Autodesk Inventor part; units mm, degrees
(part 2 of 2)
  line L262 (13.6018, -17.5742) -> (13.2961, -17.2686)
  spline S264 degree 2 poles (13.2961, -17.2686) (13.3171, -17.2092) (13.3852, -17.0328) (13.4219, -16.9716) knots 0 0 0 1 2 2 2
  spline S265 degree 2 poles (13.4219, -16.9716) (13.4708, -16.8808) (13.5599, -16.7498) (13.6454, -16.6642) knots 0 0 0 1 2 2 2
  spline S266 degree 2 poles (12.2779, -18.0318) (12.4455, -17.8641) (12.8263, -17.6895) (13.0306, -17.6947) knots 0 0 0 1 2 2 2
  spline S267 degree 2 poles (13.0306, -17.6947) (13.2332, -17.6982) (13.6612, -17.906) (13.8742, -18.1191) knots 0 0 0 1 2 2 2
  spline S268 degree 2 poles (13.8742, -18.1191) (14.0873, -18.3322) (14.2847, -18.7566) (14.2934, -18.9575) knots 0 0 0 1 2 2 2
  spline S269 degree 2 poles (14.2934, -18.9575) (14.3039, -19.1601) (14.1327, -19.5583) (13.9686, -19.7225) knots 0 0 0 1 2 2 2
  spline S270 degree 2 poles (13.9686, -19.7225) (13.8358, -19.8552) (13.5127, -20.0281) (13.3677, -20.0753) knots 0 0 0 1 2 2 2
  line L263 (13.3677, -20.0753) -> (13.0621, -19.7696)
  line L264 (13.0621, -19.7696) -> (13.0778, -19.7539)
  spline S271 degree 2 poles (13.0778, -19.7539) (13.1319, -19.7487) (13.2856, -19.7207) (13.3835, -19.6893) knots 0 0 0 1 2 2 2
  spline S272 degree 2 poles (13.3835, -19.6893) (13.469, -19.6596) (13.6664, -19.5496) (13.7363, -19.4797) knots 0 0 0 1 2 2 2
  spline S273 degree 2 poles (13.7363, -19.4797) (13.9476, -19.2684) (13.8847, -18.692) (13.593, -18.4003) knots 0 0 0 1 2 2 2
  spline S274 degree 2 poles (13.593, -18.4003) (13.3084, -18.1156) (12.7407, -18.044) (12.5207, -18.2641) knots 0 0 0 1 2 2 2
  spline S275 degree 2 poles (12.5207, -18.2641) (12.3879, -18.3968) (12.2569, -18.7479) (12.2499, -18.926) knots 0 0 0 1 2 2 2
  line L265 (12.2499, -18.926) -> (12.2342, -18.9418)
  line L266 (12.2342, -18.9418) -> (11.9286, -18.6361)
  spline S276 degree 2 poles (11.9286, -18.6361) (11.9495, -18.5767) (12.0176, -18.4003) (12.0543, -18.3392) knots 0 0 0 1 2 2 2
  spline S277 degree 2 poles (12.0543, -18.3392) (12.1032, -18.2484) (12.1923, -18.1174) (12.2779, -18.0318) knots 0 0 0 1 2 2 2
  line L267 (11.312, -19.071) -> (11.5845, -18.7985)
  line L268 (11.5845, -18.7985) -> (13.2018, -20.4159)
  line L269 (13.2018, -20.4159) -> (12.9293, -20.6883)
  line L270 (12.9293, -20.6883) -> (11.312, -19.071)
  line L271 (13.1791, -20.9765) -> (13.4882, -20.6674)
  line L272 (13.4882, -20.6674) -> (13.7712, -20.9503)
  line L273 (13.7712, -20.9503) -> (13.462, -21.2595)
  line L274 (13.462, -21.2595) -> (13.1791, -20.9765)
  spline S278 degree 2 poles (10.3916, -21.6088) (9.9829, -21.2001) (9.9305, -20.3617) (10.2588, -20.0334) knots 0 0 0 1 2 2 2
  spline S279 degree 2 poles (10.2588, -20.0334) (10.5959, -19.6963) (11.4413, -19.7696) (11.836, -20.1644) knots 0 0 0 1 2 2 2
  spline S280 degree 2 poles (11.836, -20.1644) (12.2412, -20.5696) (12.2919, -21.4166) (11.967, -21.7415) knots 0 0 0 1 2 2 2
  spline S281 degree 2 poles (11.967, -21.7415) (11.6386, -22.0699) (10.7985, -22.0157) (10.3916, -21.6088) knots 0 0 0 1 2 2 2
  spline S282 degree 2 poles (10.6728, -21.3276) (10.9872, -21.642) (11.5216, -21.7188) (11.7329, -21.5075) knots 0 0 0 1 2 2 2
  spline S283 degree 2 poles (11.7329, -21.5075) (11.9443, -21.2961) (11.8692, -20.7599) (11.5548, -20.4456) knots 0 0 0 1 2 2 2
  spline S284 degree 2 poles (11.5548, -20.4456) (11.2492, -20.1399) (10.7042, -20.0561) (10.4929, -20.2674) knots 0 0 0 1 2 2 2
  spline S285 degree 2 poles (10.4929, -20.2674) (10.2833, -20.477) (10.3619, -21.0167) (10.6728, -21.3276) knots 0 0 0 1 2 2 2
  line L275 (14.7087, -8.5772) -> (15.9575, -7.3284)
  line L276 (15.9575, -7.3284) -> (18.1127, -9.4837)
  line L277 (18.1127, -9.4837) -> (17.8263, -9.7701)
  line L278 (17.8263, -9.7701) -> (15.926, -7.8699)
  line L279 (15.926, -7.8699) -> (14.9637, -8.8322)
  line L280 (14.9637, -8.8322) -> (14.7087, -8.5772)
  spline S286 degree 2 poles (13.7655, -9.447) (14.1533, -9.0593) (15.0143, -9.068) (15.416, -9.4697) knots 0 0 0 1 2 2 2
  spline S287 degree 2 poles (15.416, -9.4697) (15.8107, -9.8644) (15.8649, -10.7464) (15.5313, -11.08) knots 0 0 0 1 2 2 2
  spline S288 degree 2 poles (15.5313, -11.08) (15.3811, -11.2302) (15.0615, -11.3752) (14.8833, -11.3682) knots 0 0 0 1 2 2 2
  spline S289 degree 2 poles (14.8833, -11.3682) (14.7034, -11.363) (14.3436, -11.1883) (14.1498, -10.9945) knots 0 0 0 1 2 2 2
  line L281 (14.1498, -10.9945) -> (14.0013, -10.846)
  line L282 (14.0013, -10.846) -> (15.1209, -9.7265)
  spline S290 degree 2 poles (15.1209, -9.7265) (14.8397, -9.4453) (14.258, -9.4295) (14.0065, -9.681) knots 0 0 0 1 2 2 2
  spline S291 degree 2 poles (14.0065, -9.681) (13.9175, -9.7701) (13.7847, -9.9832) (13.7463, -10.0845) knots 0 0 0 1 2 2 2
  spline S292 degree 2 poles (13.7463, -10.0845) (13.7079, -10.1928) (13.6677, -10.3552) (13.6625, -10.4163) knots 0 0 0 1 2 2 2
  line L283 (13.6625, -10.4163) -> (13.6468, -10.4321)
  line L284 (13.6468, -10.4321) -> (13.3498, -10.1351)
  spline S293 degree 2 poles (13.3498, -10.1351) (13.3778, -10.0688) (13.4651, -9.8697) (13.5053, -9.7981) knots 0 0 0 1 2 2 2
  spline S294 degree 2 poles (13.5053, -9.7981) (13.5612, -9.6968) (13.6677, -9.5448) (13.7655, -9.447) knots 0 0 0 1 2 2 2
  spline S295 degree 2 poles (14.4746, -10.7884) (14.5881, -10.8949) (14.7942, -11.0102) (14.8921, -11.0207) knots 0 0 0 1 2 2 2
  spline S296 degree 2 poles (14.8921, -11.0207) (15.0003, -11.0346) (15.2134, -10.9508) (15.3235, -10.8408) knots 0 0 0 1 2 2 2
  spline S297 degree 2 poles (15.3235, -10.8408) (15.4317, -10.7325) (15.5191, -10.5159) (15.5191, -10.3901) knots 0 0 0 1 2 2 2
  spline S298 degree 2 poles (15.5191, -10.3901) (15.5156, -10.2644) (15.423, -10.0461) (15.3287, -9.9343) knots 0 0 0 1 2 2 2
  line L285 (15.3287, -9.9343) -> (14.4746, -10.7884)
  spline S299 degree 2 poles (12.4242, -12.479) (12.0155, -12.0703) (11.9631, -11.232) (12.2914, -10.9036) knots 0 0 0 1 2 2 2
  spline S300 degree 2 poles (12.2914, -10.9036) (12.6285, -10.5665) (13.4738, -10.6399) (13.8686, -11.0346) knots 0 0 0 1 2 2 2
  spline S301 degree 2 poles (13.8686, -11.0346) (14.2738, -11.4398) (14.3244, -12.2869) (13.9996, -12.6118) knots 0 0 0 1 2 2 2
  spline S302 degree 2 poles (13.9996, -12.6118) (13.6712, -12.9401) (12.8311, -12.886) (12.4242, -12.479) knots 0 0 0 1 2 2 2
  spline S303 degree 2 poles (12.7054, -12.1978) (13.0197, -12.5122) (13.5542, -12.5891) (13.7655, -12.3777) knots 0 0 0 1 2 2 2
  spline S304 degree 2 poles (13.7655, -12.3777) (13.9769, -12.1664) (13.9017, -11.6302) (13.5874, -11.3158) knots 0 0 0 1 2 2 2
  spline S305 degree 2 poles (13.5874, -11.3158) (13.2817, -11.0102) (12.7368, -10.9263) (12.5255, -11.1377) knots 0 0 0 1 2 2 2
  spline S306 degree 2 poles (12.5255, -11.1377) (12.3159, -11.3473) (12.3945, -11.887) (12.7054, -12.1978) knots 0 0 0 1 2 2 2
  line L286 (10.0663, -13.2196) -> (10.3388, -12.9471)
  line L287 (10.3388, -12.9471) -> (11.2609, -13.8693)
  spline S307 degree 2 poles (11.2609, -13.8693) (11.3727, -13.9811) (11.5858, -14.1522) (11.6749, -14.1784) knots 0 0 0 1 2 2 2
  spline S308 degree 2 poles (11.6749, -14.1784) (11.7692, -14.2064) (11.9473, -14.147) (12.0486, -14.0457) knots 0 0 0 1 2 2 2
  spline S309 degree 2 poles (12.0486, -14.0457) (12.1499, -13.9444) (12.2565, -13.6213) (12.2722, -13.4309) knots 0 0 0 1 2 2 2
  line L288 (12.2722, -13.4309) -> (11.0636, -12.2223)
  line L289 (11.0636, -12.2223) -> (11.336, -11.9498)
  line L290 (11.336, -11.9498) -> (12.9534, -13.5671)
  line L291 (12.9534, -13.5671) -> (12.6809, -13.8396)
  line L292 (12.6809, -13.8396) -> (12.501, -13.6597)
  spline S310 degree 2 poles (12.501, -13.6597) (12.4888, -13.892) (12.3683, -14.2431) (12.2355, -14.3758) knots 0 0 0 1 2 2 2
  spline S311 degree 2 poles (12.2355, -14.3758) (11.998, -14.6133) (11.4146, -14.5679) (11.116, -14.2693) knots 0 0 0 1 2 2 2
  line L293 (11.116, -14.2693) -> (10.0663, -13.2196)
  spline S312 degree 2 poles (8.9537, -14.6745) (8.9625, -14.6168) (8.9869, -14.4177) (9.0131, -14.3391) knots 0 0 0 1 2 2 2
  spline S313 degree 2 poles (9.0131, -14.3391) (9.0463, -14.2291) (9.1406, -14.0544) (9.2629, -13.9322) knots 0 0 0 1 2 2 2
  spline S314 degree 2 poles (9.2629, -13.9322) (9.3624, -13.8326) (9.6174, -13.7278) (9.7537, -13.7278) knots 0 0 0 1 2 2 2
  spline S315 degree 2 poles (9.7537, -13.7278) (9.8846, -13.7296) (10.1589, -13.8466) (10.2671, -13.9549) knots 0 0 0 1 2 2 2
  spline S316 degree 2 poles (10.2671, -13.9549) (10.4348, -14.1226) (10.5309, -14.5016) (10.4453, -14.7234) knots 0 0 0 1 2 2 2
  spline S317 degree 2 poles (10.4453, -14.7234) (10.3719, -14.9225) (10.0488, -15.3399) (9.8462, -15.567) knots 0 0 0 1 2 2 2
  line L294 (9.8462, -15.567) -> (9.8986, -15.6194)
  spline S318 degree 2 poles (9.8986, -15.6194) (9.9929, -15.7137) (10.1676, -15.7731) (10.2532, -15.7538) knots 0 0 0 1 2 2 2
  spline S319 degree 2 poles (10.2532, -15.7538) (10.3388, -15.7346) (10.5099, -15.6054) (10.5903, -15.525) knots 0 0 0 1 2 2 2
  spline S320 degree 2 poles (10.5903, -15.525) (10.6846, -15.4307) (10.8837, -15.1198) (10.957, -14.9382) knots 0 0 0 1 2 2 2
  line L295 (10.957, -14.9382) -> (10.9728, -14.9225)
  line L296 (10.9728, -14.9225) -> (11.2505, -15.2002)
  spline S321 degree 2 poles (11.2505, -15.2002) (11.1963, -15.2962) (10.9675, -15.6298) (10.8295, -15.7678) knots 0 0 0 1 2 2 2
  spline S322 degree 2 poles (10.8295, -15.7678) (10.6619, -15.9355) (10.3807, -16.1119) (10.2217, -16.1346) knots 0 0 0 1 2 2 2
  spline S323 degree 2 poles (10.2217, -16.1346) (10.0663, -16.1573) (9.7676, -16.0333) (9.6157, -15.8813) knots 0 0 0 1 2 2 2
  line L297 (9.6157, -15.8813) -> (8.5101, -14.7758)
  line L298 (8.5101, -14.7758) -> (8.7826, -14.5033)
  line L299 (8.7826, -14.5033) -> (8.9537, -14.6745)
  line L300 (9.1808, -14.9015) -> (9.6297, -15.3504)
  spline S324 degree 2 poles (9.6297, -15.3504) (9.7187, -15.2439) (9.9842, -14.919) (10.0488, -14.7985) knots 0 0 0 1 2 2 2
  spline S325 degree 2 poles (10.0488, -14.7985) (10.1239, -14.657) (10.1274, -14.3776) (10.0052, -14.2553) knots 0 0 0 1 2 2 2
  spline S326 degree 2 poles (10.0052, -14.2553) (9.8654, -14.1156) (9.5668, -14.1313) (9.4166, -14.2815) knots 0 0 0 1 2 2 2
  spline S327 degree 2 poles (9.4166, -14.2815) (9.2891, -14.409) (9.1895, -14.7286) (9.1808, -14.9015) knots 0 0 0 1 2 2 2
  line L301 (8.5957, -17.3415) -> (8.6097, -17.3275)
  spline S328 degree 2 poles (8.6097, -17.3275) (8.6498, -17.3048) (8.7214, -17.2402) (8.7686, -17.193) knots 0 0 0 1 2 2 2
  spline S329 degree 2 poles (8.7686, -17.193) (8.8786, -17.083) (8.9991, -16.7703) (9.0026, -16.5782) knots 0 0 0 1 2 2 2
  line L302 (9.0026, -16.5782) -> (7.8551, -15.4307)
  line L303 (7.8551, -15.4307) -> (8.1276, -15.1583)
  line L304 (8.1276, -15.1583) -> (9.7449, -16.7756)
  line L305 (9.7449, -16.7756) -> (9.4725, -17.0481)
  line L306 (9.4725, -17.0481) -> (9.2314, -16.807)
  spline S330 degree 2 poles (9.2314, -16.807) (9.2157, -17.0882) (9.1022, -17.4183) (8.9974, -17.5231) knots 0 0 0 1 2 2 2
  spline S331 degree 2 poles (8.9974, -17.5231) (8.9555, -17.565) (8.9101, -17.6035) (8.8786, -17.6244) knots 0 0 0 1 2 2 2
  line L307 (8.8786, -17.6244) -> (8.5957, -17.3415)
  line L308 (5.8152, -17.4707) -> (6.0876, -17.1983)
  line L309 (6.0876, -17.1983) -> (6.2518, -17.3624)
  spline S332 degree 2 poles (6.2518, -17.3624) (6.2623, -17.2472) (6.285, -17.0847) (6.3182, -16.9922) knots 0 0 0 1 2 2 2
  spline S333 degree 2 poles (6.3182, -16.9922) (6.3479, -16.9066) (6.4422, -16.7529) (6.5243, -16.6708) knots 0 0 0 1 2 2 2
  spline S334 degree 2 poles (6.5243, -16.6708) (6.657, -16.5381) (6.9906, -16.4245) (7.1757, -16.4525) knots 0 0 0 1 2 2 2
  spline S335 degree 2 poles (7.1757, -16.4525) (7.3609, -16.4804) (7.7626, -16.7075) (7.9669, -16.9118) knots 0 0 0 1 2 2 2
  spline S336 degree 2 poles (7.9669, -16.9118) (8.18, -17.1249) (8.3809, -17.5458) (8.4018, -17.7589) knots 0 0 0 1 2 2 2
  spline S337 degree 2 poles (8.4018, -17.7589) (8.4175, -17.9528) (8.2883, -18.323) (8.1503, -18.461) knots 0 0 0 1 2 2 2
  spline S338 degree 2 poles (8.1503, -18.461) (8.0298, -18.5815) (7.7958, -18.7073) (7.6403, -18.751) knots 0 0 0 1 2 2 2
  line L310 (7.6403, -18.751) -> (8.3389, -19.4496)
  line L311 (8.3389, -19.4496) -> (8.0665, -19.722)
  line L312 (8.0665, -19.722) -> (5.8152, -17.4707)
  line L313 (6.4806, -17.5912) -> (7.415, -18.5256)
  spline S339 degree 2 poles (7.415, -18.5256) (7.5652, -18.4732) (7.7626, -18.3492) (7.8551, -18.2567) knots 0 0 0 1 2 2 2
  spline S340 degree 2 poles (7.8551, -18.2567) (8.0647, -18.0471) (7.9879, -17.4952) (7.691, -17.1983) knots 0 0 0 1 2 2 2
  spline S341 degree 2 poles (7.691, -17.1983) (7.4045, -16.9118) (6.9207, -16.7913) (6.7199, -16.9922) knots 0 0 0 1 2 2 2
  spline S342 degree 2 poles (6.7199, -16.9922) (6.6133, -17.0987) (6.4946, -17.4131) (6.4806, -17.5912) knots 0 0 0 1 2 2 2
  spline S343 degree 2 poles (4.9, -20.0032) (4.4913, -19.5945) (4.4389, -18.7562) (4.7672, -18.4278) knots 0 0 0 1 2 2 2
  spline S344 degree 2 poles (4.7672, -18.4278) (5.1043, -18.0908) (5.9496, -18.1641) (6.3444, -18.5588) knots 0 0 0 1 2 2 2
  spline S345 degree 2 poles (6.3444, -18.5588) (6.7496, -18.964) (6.8002, -19.8111) (6.4754, -20.136) knots 0 0 0 1 2 2 2
  spline S346 degree 2 poles (6.4754, -20.136) (6.147, -20.4643) (5.3069, -20.4102) (4.9, -20.0032) knots 0 0 0 1 2 2 2
  spline S347 degree 2 poles (5.1811, -19.722) (5.4955, -20.0364) (6.03, -20.1133) (6.2413, -19.9019) knots 0 0 0 1 2 2 2
  spline S348 degree 2 poles (6.2413, -19.9019) (6.4526, -19.6906) (6.3775, -19.1544) (6.0632, -18.84) knots 0 0 0 1 2 2 2
  spline S349 degree 2 poles (6.0632, -18.84) (5.7575, -18.5344) (5.2126, -18.4505) (5.0013, -18.6619) knots 0 0 0 1 2 2 2
  spline S350 degree 2 poles (5.0013, -18.6619) (4.7917, -18.8715) (4.8703, -19.4112) (5.1811, -19.722) knots 0 0 0 1 2 2 2
  line L314 (-17.3745, -18.836) -> (-14.477, -17.4231)
  line L315 (-14.477, -17.4231) -> (-14.1679, -17.7322)
  line L316 (-14.1679, -17.7322) -> (-15.5808, -20.6297)
  line L317 (-15.5808, -20.6297) -> (-15.8882, -20.3224)
  line L318 (-15.8882, -20.3224) -> (-14.6953, -17.9348)
  line L319 (-14.6953, -17.9348) -> (-17.0829, -19.1277)
  line L320 (-17.0829, -19.1277) -> (-17.3745, -18.836)
  line L321 (-15.6821, -16.2179) -> (-15.4097, -16.4904)
  line L322 (-15.4097, -16.4904) -> (-17.027, -18.1077)
  line L323 (-17.027, -18.1077) -> (-17.2994, -17.8352)
  line L324 (-17.2994, -17.8352) -> (-15.6821, -16.2179)
  line L325 (-17.5876, -18.085) -> (-17.2785, -18.3941)
  line L326 (-17.2785, -18.3941) -> (-17.5614, -18.6771)
  line L327 (-17.5614, -18.6771) -> (-17.8706, -18.3679)
  line L328 (-17.8706, -18.3679) -> (-17.5876, -18.085)
  spline S351 degree 2 poles (-16.5397, -15.2975) (-16.3179, -15.5193) (-16.3214, -16.0223) (-16.5956, -16.2965) knots 0 0 0 1 2 2 2
  line L329 (-16.5956, -16.2965) -> (-17.4916, -17.1925)
  line L330 (-17.4916, -17.1925) -> (-17.3082, -17.3759)
  line L331 (-17.3082, -17.3759) -> (-17.5335, -17.6012)
  line L332 (-17.5335, -17.6012) -> (-17.7169, -17.4178)
  line L333 (-17.7169, -17.4178) -> (-18.1815, -17.8824)
  line L334 (-18.1815, -17.8824) -> (-18.4539, -17.6099)
  line L335 (-18.4539, -17.6099) -> (-17.9893, -17.1454)
  line L336 (-17.9893, -17.1454) -> (-18.4906, -16.6441)
  line L337 (-18.4906, -16.6441) -> (-18.2653, -16.4188)
  line L338 (-18.2653, -16.4188) -> (-17.764, -16.92)
  line L339 (-17.764, -16.92) -> (-16.9938, -16.1498)
  spline S352 degree 2 poles (-16.9938, -16.1498) (-16.8715, -16.0275) (-16.7458, -15.8843) (-16.7178, -15.797) knots 0 0 0 1 2 2 2
  spline S353 degree 2 poles (-16.7178, -15.797) (-16.6916, -15.7219) (-16.751, -15.5612) (-16.8453, -15.4669) knots 0 0 0 1 2 2 2
  spline S354 degree 2 poles (-16.8453, -15.4669) (-16.9117, -15.4005) (-17.0759, -15.3167) (-17.1161, -15.301) knots 0 0 0 1 2 2 2
  line L340 (-17.1161, -15.301) -> (-17.1318, -15.2853)
  line L341 (-17.1318, -15.2853) -> (-16.8873, -15.0407)
  spline S355 degree 2 poles (-16.8873, -15.0407) (-16.7894, -15.0966) (-16.6078, -15.2294) (-16.5397, -15.2975) knots 0 0 0 1 2 2 2
  spline S356 degree 2 poles (-17.5317, -14.3054) (-17.3099, -14.5272) (-17.3134, -15.0303) (-17.5876, -15.3045) knots 0 0 0 1 2 2 2
  line L342 (-17.5876, -15.3045) -> (-18.4836, -16.2005)
  line L343 (-18.4836, -16.2005) -> (-18.3002, -16.3838)
  line L344 (-18.3002, -16.3838) -> (-18.5255, -16.6092)
  line L345 (-18.5255, -16.6092) -> (-18.7089, -16.4258)
  line L346 (-18.7089, -16.4258) -> (-19.1735, -16.8904)
  line L347 (-19.1735, -16.8904) -> (-19.446, -16.6179)
  line L348 (-19.446, -16.6179) -> (-18.9814, -16.1533)
  line L349 (-18.9814, -16.1533) -> (-19.4827, -15.652)
  line L350 (-19.4827, -15.652) -> (-19.2573, -15.4267)
  line L351 (-19.2573, -15.4267) -> (-18.7561, -15.928)
  line L352 (-18.7561, -15.928) -> (-17.9858, -15.1578)
  spline S357 degree 2 poles (-17.9858, -15.1578) (-17.8636, -15.0355) (-17.7378, -14.8923) (-17.7099, -14.805) knots 0 0 0 1 2 2 2
  spline S358 degree 2 poles (-17.7099, -14.805) (-17.6837, -14.7299) (-17.7431, -14.5692) (-17.8374, -14.4749) knots 0 0 0 1 2 2 2
  spline S359 degree 2 poles (-17.8374, -14.4749) (-17.9038, -14.4085) (-18.0679, -14.3246) (-18.1081, -14.3089) knots 0 0 0 1 2 2 2
  line L353 (-18.1081, -14.3089) -> (-18.1238, -14.2932)
  line L354 (-18.1238, -14.2932) -> (-17.8793, -14.0487)
  spline S360 degree 2 poles (-17.8793, -14.0487) (-17.7815, -14.1046) (-17.5999, -14.2373) (-17.5317, -14.3054) knots 0 0 0 1 2 2 2
  line L355 (-18.3439, -13.5562) -> (-18.0714, -13.8286)
  line L356 (-18.0714, -13.8286) -> (-19.6887, -15.4459)
  line L357 (-19.6887, -15.4459) -> (-19.9612, -15.1735)
  line L358 (-19.9612, -15.1735) -> (-18.3439, -13.5562)
  line L359 (-20.2494, -15.4232) -> (-19.9403, -15.7324)
  line L360 (-19.9403, -15.7324) -> (-20.2232, -16.0153)
  line L361 (-20.2232, -16.0153) -> (-20.5323, -15.7062)
  line L362 (-20.5323, -15.7062) -> (-20.2494, -15.4232)
  spline S361 degree 2 poles (-8.1645, -16.5546) (-7.9357, -16.7834) (-7.6964, -17.3021) (-7.7016, -17.5798) knots 0 0 0 1 2 2 2
  spline S362 degree 2 poles (-7.7016, -17.5798) (-7.7086, -17.8593) (-7.9863, -18.4269) (-8.2605, -18.7011) knots 0 0 0 1 2 2 2
  spline S363 degree 2 poles (-8.2605, -18.7011) (-8.5208, -18.9613) (-9.0797, -19.2268) (-9.3626, -19.2373) knots 0 0 0 1 2 2 2
  spline S364 degree 2 poles (-9.3626, -19.2373) (-9.6351, -19.2478) (-10.173, -19.0172) (-10.4018, -18.7884) knots 0 0 0 1 2 2 2
  spline S365 degree 2 poles (-10.4018, -18.7884) (-10.5119, -18.6784) (-10.6795, -18.4479) (-10.7424, -18.3291) knots 0 0 0 1 2 2 2
  spline S366 degree 2 poles (-10.7424, -18.3291) (-10.7948, -18.2348) (-10.8961, -17.9798) (-10.9223, -17.8977) knots 0 0 0 1 2 2 2
  line L363 (-10.9223, -17.8977) -> (-10.5765, -17.5519)
  line L364 (-10.5765, -17.5519) -> (-10.552, -17.5763)
  spline S367 degree 2 poles (-10.552, -17.5763) (-10.545, -17.6776) (-10.5171, -17.8767) (-10.4612, -18.0304) knots 0 0 0 1 2 2 2
  spline S368 degree 2 poles (-10.4612, -18.0304) (-10.4175, -18.1614) (-10.2499, -18.4444) (-10.1206, -18.5736) knots 0 0 0 1 2 2 2
  spline S369 degree 2 poles (-10.1206, -18.5736) (-9.8097, -18.8845) (-8.9574, -18.8007) (-8.5679, -18.4112) knots 0 0 0 1 2 2 2
  spline S370 degree 2 poles (-8.5679, -18.4112) (-8.3514, -18.1946) (-8.1278, -17.7684) (-8.1121, -17.5606) knots 0 0 0 1 2 2 2
  spline S371 degree 2 poles (-8.1121, -17.5606) (-8.0929, -17.3563) (-8.2378, -16.9772) (-8.402, -16.8131) knots 0 0 0 1 2 2 2
  spline S372 degree 2 poles (-8.402, -16.8131) (-8.5225, -16.6926) (-8.7985, -16.4865) (-8.9155, -16.4393) knots 0 0 0 1 2 2 2
  line L365 (-8.9155, -16.4393) -> (-9.4727, -16.9965)
  line L366 (-9.4727, -16.9965) -> (-8.9731, -17.496)
  line L367 (-8.9731, -17.496) -> (-9.2246, -17.7475)
  line L368 (-9.2246, -17.7475) -> (-10.0071, -16.965)
  line L369 (-10.0071, -16.965) -> (-9.0657, -16.0236)
  spline S373 degree 2 poles (-9.0657, -16.0236) (-8.9871, -16.0533) (-8.7269, -16.1633) (-8.6256, -16.2192) knots 0 0 0 1 2 2 2
  spline S374 degree 2 poles (-8.6256, -16.2192) (-8.4876, -16.2943) (-8.285, -16.4341) (-8.1645, -16.5546) knots 0 0 0 1 2 2 2
  spline S375 degree 2 poles (-10.3337, -14.8115) (-10.2761, -14.8202) (-10.077, -14.8447) (-9.9984, -14.8709) knots 0 0 0 1 2 2 2
  spline S376 degree 2 poles (-9.9984, -14.8709) (-9.8883, -14.9041) (-9.7137, -14.9984) (-9.5914, -15.1206) knots 0 0 0 1 2 2 2
  spline S377 degree 2 poles (-9.5914, -15.1206) (-9.4919, -15.2202) (-9.3871, -15.4752) (-9.3871, -15.6114) knots 0 0 0 1 2 2 2
  spline S378 degree 2 poles (-9.3871, -15.6114) (-9.3888, -15.7424) (-9.5058, -16.0166) (-9.6141, -16.1249) knots 0 0 0 1 2 2 2
  spline S379 degree 2 poles (-9.6141, -16.1249) (-9.7818, -16.2926) (-10.1608, -16.3887) (-10.3826, -16.3031) knots 0 0 0 1 2 2 2
  spline S380 degree 2 poles (-10.3826, -16.3031) (-10.5817, -16.2297) (-10.9992, -15.9066) (-11.2262, -15.704) knots 0 0 0 1 2 2 2
  line L370 (-11.2262, -15.704) -> (-11.2786, -15.7564)
  spline S381 degree 2 poles (-11.2786, -15.7564) (-11.3729, -15.8507) (-11.4323, -16.0254) (-11.4131, -16.111) knots 0 0 0 1 2 2 2
  spline S382 degree 2 poles (-11.4131, -16.111) (-11.3939, -16.1965) (-11.2646, -16.3677) (-11.1843, -16.448) knots 0 0 0 1 2 2 2
  spline S383 degree 2 poles (-11.1843, -16.448) (-11.09, -16.5424) (-10.7791, -16.7415) (-10.5974, -16.8148) knots 0 0 0 1 2 2 2
  line L371 (-10.5974, -16.8148) -> (-10.5817, -16.8305)
  line L372 (-10.5817, -16.8305) -> (-10.8594, -17.1082)
  spline S384 degree 2 poles (-10.8594, -17.1082) (-10.9555, -17.0541) (-11.2891, -16.8253) (-11.4271, -16.6873) knots 0 0 0 1 2 2 2
  spline S385 degree 2 poles (-11.4271, -16.6873) (-11.5947, -16.5196) (-11.7711, -16.2384) (-11.7938, -16.0795) knots 0 0 0 1 2 2 2
  spline S386 degree 2 poles (-11.7938, -16.0795) (-11.8165, -15.9241) (-11.6925, -15.6254) (-11.5406, -15.4735) knots 0 0 0 1 2 2 2
  line L373 (-11.5406, -15.4735) -> (-10.435, -14.3679)
  line L374 (-10.435, -14.3679) -> (-10.1625, -14.6403)
  line L375 (-10.1625, -14.6403) -> (-10.3337, -14.8115)
  line L376 (-10.5608, -15.0386) -> (-11.0096, -15.4874)
  spline S387 degree 2 poles (-11.0096, -15.4874) (-10.9031, -15.5765) (-10.5782, -15.842) (-10.4577, -15.9066) knots 0 0 0 1 2 2 2
  spline S388 degree 2 poles (-10.4577, -15.9066) (-10.3162, -15.9817) (-10.0368, -15.9852) (-9.9145, -15.8629) knots 0 0 0 1 2 2 2
  spline S389 degree 2 poles (-9.9145, -15.8629) (-9.7748, -15.7232) (-9.7905, -15.4246) (-9.9407, -15.2743) knots 0 0 0 1 2 2 2
  spline S390 degree 2 poles (-9.9407, -15.2743) (-10.0682, -15.1468) (-10.3879, -15.0473) (-10.5608, -15.0386) knots 0 0 0 1 2 2 2
  spline S391 degree 2 poles (-13.0077, -13.4649) (-12.6112, -13.0684) (-11.7432, -12.9689) (-11.4533, -13.2588) knots 0 0 0 1 2 2 2
  spline S392 degree 2 poles (-11.4533, -13.2588) (-11.3223, -13.3898) (-11.2, -13.6413) (-11.1651, -13.788) knots 0 0 0 1 2 2 2
  line L377 (-11.1651, -13.788) -> (-11.0725, -13.7304)
  line L378 (-11.0725, -13.7304) -> (-10.8175, -13.9854)
  line L379 (-10.8175, -13.9854) -> (-13.0688, -16.2367)
  line L380 (-13.0688, -16.2367) -> (-13.3413, -15.9642)
  line L381 (-13.3413, -15.9642) -> (-12.5379, -15.1608)
  spline S393 degree 2 poles (-12.5379, -15.1608) (-12.7335, -15.1503) (-13.095, -15.0333) (-13.247, -14.8814) knots 0 0 0 1 2 2 2
  spline S394 degree 2 poles (-13.247, -14.8814) (-13.5212, -14.6072) (-13.3972, -13.8544) (-13.0077, -13.4649) knots 0 0 0 1 2 2 2
  spline S395 degree 2 poles (-12.7055, -13.7251) (-12.9955, -14.0151) (-13.1195, -14.4919) (-12.9239, -14.6875) knots 0 0 0 1 2 2 2
  spline S396 degree 2 poles (-12.9239, -14.6875) (-12.8138, -14.7975) (-12.482, -14.9198) (-12.3091, -14.932) knots 0 0 0 1 2 2 2
  line L382 (-12.3091, -14.932) -> (-11.3816, -14.0046)
  spline S397 degree 2 poles (-11.3816, -14.0046) (-11.434, -13.8509) (-11.5511, -13.65) (-11.6454, -13.5557) knots 0 0 0 1 2 2 2
  spline S398 degree 2 poles (-11.6454, -13.5557) (-11.8532, -13.3479) (-12.3859, -13.4055) (-12.7055, -13.7251) knots 0 0 0 1 2 2 2
  line L383 (-14.639, -12.8152) -> (-14.625, -12.8292)
  spline S399 degree 2 poles (-14.625, -12.8292) (-14.6023, -12.8693) (-14.5377, -12.9409) (-14.4905, -12.9881) knots 0 0 0 1 2 2 2
  spline S400 degree 2 poles (-14.4905, -12.9881) (-14.3805, -13.0981) (-14.0679, -13.2186) (-13.8757, -13.2221) knots 0 0 0 1 2 2 2
  line L384 (-13.8757, -13.2221) -> (-12.7283, -12.0746)
  line L385 (-12.7283, -12.0746) -> (-12.4558, -12.3471)
  line L386 (-12.4558, -12.3471) -> (-14.0731, -13.9644)
  line L387 (-14.0731, -13.9644) -> (-14.3456, -13.692)
  line L388 (-14.3456, -13.692) -> (-14.1045, -13.4509)
  spline S401 degree 2 poles (-14.1045, -13.4509) (-14.3857, -13.4352) (-14.7158, -13.3217) (-14.8206, -13.2169) knots 0 0 0 1 2 2 2
  spline S402 degree 2 poles (-14.8206, -13.2169) (-14.8626, -13.175) (-14.901, -13.1296) (-14.9219, -13.0981) knots 0 0 0 1 2 2 2
  line L389 (-14.9219, -13.0981) -> (-14.639, -12.8152)
  line L390 (-13.8024, -11.0005) -> (-13.5299, -11.273)
  line L391 (-13.5299, -11.273) -> (-15.1472, -12.8903)
  line L392 (-15.1472, -12.8903) -> (-15.4197, -12.6178)
  line L393 (-15.4197, -12.6178) -> (-13.8024, -11.0005)
  line L394 (-15.7079, -12.8676) -> (-15.3987, -13.1767)
  line L395 (-15.3987, -13.1767) -> (-15.6817, -13.4597)
  line L396 (-15.6817, -13.4597) -> (-15.9908, -13.1505)
  line L397 (-15.9908, -13.1505) -> (-15.7079, -12.8676)
  spline S403 degree 2 poles (-14.8678, -9.8617) (-14.4801, -10.2495) (-14.4888, -11.1105) (-14.8905, -11.5122) knots 0 0 0 1 2 2 2
  spline S404 degree 2 poles (-14.8905, -11.5122) (-15.2852, -11.907) (-16.1672, -11.9611) (-16.5008, -11.6275) knots 0 0 0 1 2 2 2
  spline S405 degree 2 poles (-16.5008, -11.6275) (-16.651, -11.4773) (-16.796, -11.1577) (-16.789, -10.9795) knots 0 0 0 1 2 2 2
  spline S406 degree 2 poles (-16.789, -10.9795) (-16.7838, -10.7996) (-16.6091, -10.4399) (-16.4152, -10.246) knots 0 0 0 1 2 2 2
  line L398 (-16.4152, -10.246) -> (-16.2668, -10.0975)
  line L399 (-16.2668, -10.0975) -> (-15.1472, -11.2171)
  spline S407 degree 2 poles (-15.1472, -11.2171) (-14.866, -10.9359) (-14.8503, -10.3543) (-15.1018, -10.1028) knots 0 0 0 1 2 2 2
  spline S408 degree 2 poles (-15.1018, -10.1028) (-15.1909, -10.0137) (-15.404, -9.881) (-15.5053, -9.8425) knots 0 0 0 1 2 2 2
  spline S409 degree 2 poles (-15.5053, -9.8425) (-15.6136, -9.8041) (-15.776, -9.7639) (-15.8371, -9.7587) knots 0 0 0 1 2 2 2
  line L400 (-15.8371, -9.7587) -> (-15.8529, -9.743)
  line L401 (-15.8529, -9.743) -> (-15.5559, -9.4461)
  spline S410 degree 2 poles (-15.5559, -9.4461) (-15.4896, -9.474) (-15.2905, -9.5613) (-15.2189, -9.6015) knots 0 0 0 1 2 2 2
  spline S411 degree 2 poles (-15.2189, -9.6015) (-15.1176, -9.6574) (-14.9656, -9.7639) (-14.8678, -9.8617) knots 0 0 0 1 2 2 2
  spline S412 degree 2 poles (-16.2092, -10.5708) (-16.3157, -10.6844) (-16.431, -10.8905) (-16.4414, -10.9883) knots 0 0 0 1 2 2 2
  spline S413 degree 2 poles (-16.4414, -10.9883) (-16.4554, -11.0966) (-16.3716, -11.3096) (-16.2616, -11.4197) knots 0 0 0 1 2 2 2
  spline S414 degree 2 poles (-16.2616, -11.4197) (-16.1533, -11.528) (-15.9367, -11.6153) (-15.8109, -11.6153) knots 0 0 0 1 2 2 2
  spline S415 degree 2 poles (-15.8109, -11.6153) (-15.6852, -11.6118) (-15.4669, -11.5192) (-15.3551, -11.4249) knots 0 0 0 1 2 2 2
  line L402 (-15.3551, -11.4249) -> (-16.2092, -10.5708)
  line L403 (-16.0397, -8.7632) -> (-15.7673, -9.0356)
  line L404 (-15.7673, -9.0356) -> (-18.0186, -11.2869)
  line L405 (-18.0186, -11.2869) -> (-18.2911, -11.0145)
  line L406 (-18.2911, -11.0145) -> (-16.0397, -8.7632)
  spline S416 degree 2 poles (-17.1051, -7.6244) (-16.7174, -8.0121) (-16.7261, -8.8732) (-17.1278, -9.2749) knots 0 0 0 1 2 2 2
  spline S417 degree 2 poles (-17.1278, -9.2749) (-17.5226, -9.6696) (-18.4046, -9.7238) (-18.7382, -9.3902) knots 0 0 0 1 2 2 2
  spline S418 degree 2 poles (-18.7382, -9.3902) (-18.8884, -9.24) (-19.0334, -8.9203) (-19.0264, -8.7422) knots 0 0 0 1 2 2 2
  spline S419 degree 2 poles (-19.0264, -8.7422) (-19.0211, -8.5623) (-18.8465, -8.2025) (-18.6526, -8.0086) knots 0 0 0 1 2 2 2
  line L407 (-18.6526, -8.0086) -> (-18.5041, -7.8602)
  line L408 (-18.5041, -7.8602) -> (-17.3846, -8.9797)
  spline S420 degree 2 poles (-17.3846, -8.9797) (-17.1034, -8.6985) (-17.0877, -8.1169) (-17.3392, -7.8654) knots 0 0 0 1 2 2 2
  spline S421 degree 2 poles (-17.3392, -7.8654) (-17.4283, -7.7763) (-17.6413, -7.6436) (-17.7426, -7.6052) knots 0 0 0 1 2 2 2
  spline S422 degree 2 poles (-17.7426, -7.6052) (-17.8509, -7.5668) (-18.0134, -7.5266) (-18.0745, -7.5213) knots 0 0 0 1 2 2 2
  line L409 (-18.0745, -7.5213) -> (-18.0902, -7.5056)
  line L410 (-18.0902, -7.5056) -> (-17.7933, -7.2087)
  spline S423 degree 2 poles (-17.7933, -7.2087) (-17.7269, -7.2367) (-17.5278, -7.324) (-17.4562, -7.3642) knots 0 0 0 1 2 2 2
  spline S424 degree 2 poles (-17.4562, -7.3642) (-17.3549, -7.42) (-17.203, -7.5266) (-17.1051, -7.6244) knots 0 0 0 1 2 2 2
  spline S425 degree 2 poles (-18.4465, -8.3335) (-18.553, -8.447) (-18.6683, -8.6531) (-18.6788, -8.7509) knots 0 0 0 1 2 2 2
  spline S426 degree 2 poles (-18.6788, -8.7509) (-18.6928, -8.8592) (-18.6089, -9.0723) (-18.4989, -9.1823) knots 0 0 0 1 2 2 2
  spline S427 degree 2 poles (-18.4989, -9.1823) (-18.3906, -9.2906) (-18.174, -9.3779) (-18.0483, -9.3779) knots 0 0 0 1 2 2 2
  spline S428 degree 2 poles (-18.0483, -9.3779) (-17.9225, -9.3744) (-17.7042, -9.2819) (-17.5924, -9.1876) knots 0 0 0 1 2 2 2
  line L411 (-17.5924, -9.1876) -> (-18.4465, -8.3335)
  dimension "d28" = 45
  dimension "d29" = 45
  dimension "d30" = 135
  dimension "d31" = 135
  constraints: 16 end point, 4 equal length, 4 horizontal, 8 other
  measures "d28" angle of L16 L17
  measures "d29" angle of L19 L18
  measures "d30" angle of L21 L20
  measures "d31" angle of L22 L23
extrude "Estrusione2" cut sketch "Schizzo4" against normal blind 1
